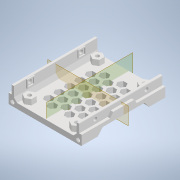
# Autodesk Inventor part: A-01
Saved by Autodesk Inventor 2022.2 (Build 262287000, 287)
## iProperties
Created: 2021-12-01
Part Number: A-01
Material: Generic
Document SubType Name: Modeling
Designer: kfcs7
Density: 1 g/cm^3
Appearance: Default
Author: kfcs7
Autodesk Inventor part; units mm, degrees
ref_plane "YZ Plane" through (0, 0, 0) normal (1, 0, 0) x (0, 1, 0)
ref_plane "XZ Plane" through (0, 0, 0) normal (0, 1, 0) x (-1, 0, 0)
ref_plane "XY Plane" through (0, 0, 0) normal (0, 0, 1) x (1, 0, 0)
sketch "Sketch1" plane through (0, 0, 0) normal (0, 1, 0) x (-1, 0, 0)
  line L0 (35, 40) -> (-35, 40)
  line L1 (-35, 40) -> (-35, -40)
  line L2 (-35, -40) -> (35, -40)
  line L3 (35, -40) -> (35, 40)
  line L4 (35, 40) -> (-35, -40) construction
  line L5 (-35, 40) -> (35, -40) construction
  point P0 (0, 0)
  dimension "d0" = 70
  dimension "d1" = 80
  constraints: 12 end point, 2 midpoint, 2 parallel, 1 horizontal, 1 perpendicular
  measures "d0" distance of L2.end L1.end
  measures "d1" distance of L1.end L0.end
extrude "Extrusion1" add sketch "Sketch1" along normal blind 17.5
chamfer "Chamfer1" distance 6 angle 45 2 edges at (35, 0, 0) (-35, 0, 0)
shell "Shell1" thickness 5 removed faces 3 at (9.6667, 11.6667, 40) at (-9.6667, 11.6667, -40) at (11.6667, 17.5, 13.3333)
ref_plane "Work Plane1" through (0, 17.5, -40) normal (-1, 0, 0) x (0, 0, 1)
ref_plane "Work Plane2" through (-29, 0, 0) normal (0, 0, 1) x (1, 0, 0)
sketch "Sketch2" plane through (-26.9289, 5, 40) normal (0, 1, 0) x (1, 0, 0)
  circle A0 centre (4.4289, 72.5) radius 1 construction
  circle A1 centre (49.4289, 72.5) radius 1 construction
  circle A2 centre (49.4289, 7.5) radius 1 construction
  circle A3 centre (4.4289, 7.5) radius 1 construction
  line L0 (1.9289, 75) -> (1.9289, 5) construction
  line L1 (1.9289, 5) -> (51.9289, 5) construction
  line L2 (51.9289, 5) -> (51.9289, 75) construction
  line L3 (51.9289, 75) -> (1.9289, 75) construction
  line L4 (4.4289, 67.3038) -> (-0.0711, 69.9019)
  line L5 (-0.0711, 69.9019) -> (-0.0711, 75.0981)
  line L6 (-0.0711, 75.0981) -> (4.4289, 77.6962)
  line L7 (4.4289, 77.6962) -> (8.9289, 75.0981)
  line L8 (8.9289, 75.0981) -> (8.9289, 69.9019)
  line L9 (8.9289, 69.9019) -> (4.4289, 67.3038)
  line L10 (44.9289, 69.9019) -> (44.9289, 75.0981)
  line L11 (44.9289, 75.0981) -> (49.4289, 77.6962)
  line L12 (49.4289, 77.6962) -> (53.9289, 75.0981)
  line L13 (53.9289, 75.0981) -> (53.9289, 69.9019)
  line L14 (53.9289, 69.9019) -> (49.4289, 67.3038)
  line L15 (49.4289, 67.3038) -> (44.9289, 69.9019)
  line L16 (4.4289, 12.6962) -> (8.9289, 10.0981)
  line L17 (8.9289, 10.0981) -> (8.9289, 4.9019)
  line L18 (8.9289, 4.9019) -> (4.4289, 2.3038)
  line L19 (4.4289, 2.3038) -> (-0.0711, 4.9019)
  line L20 (-0.0711, 4.9019) -> (-0.0711, 10.0981)
  line L21 (-0.0711, 10.0981) -> (4.4289, 12.6962)
  line L22 (44.9289, 10.0981) -> (49.4289, 12.6962)
  line L23 (49.4289, 12.6962) -> (53.9289, 10.0981)
  line L24 (53.9289, 10.0981) -> (53.9289, 4.9019)
  line L25 (53.9289, 4.9019) -> (49.4289, 2.3038)
  line L26 (49.4289, 2.3038) -> (44.9289, 4.9019)
  line L27 (44.9289, 4.9019) -> (44.9289, 10.0981)
  circle A4 centre (4.4289, 72.5) radius 1.25
  circle A5 centre (4.4289, 7.5) radius 1.25
  circle A6 centre (49.4289, 7.5) radius 1.25
  circle A7 centre (49.4289, 72.5) radius 1.25
  point P0 (26.9289, 40)
  dimension "d8" = 2.5
  dimension "d9" = 9
  dimension "d10" = 9
  dimension "d11" = 9
  dimension "d12" = 9
  dimension "d13" = 2.5
  dimension "d14" = 2.5
  dimension "d15" = 2.5
  constraints: 48 end point, 8 coincident, 4 centre point, 4 parallel, 52 other
  measures "d8" diameter of A4
  measures "d9" distance between parallel lines of L8 L5
  measures "d10" distance between parallel lines of L13 L10
  measures "d11" distance between parallel lines of L24 L27
  measures "d12" distance between parallel lines of L17 L20
  measures "d13" diameter of A5
  measures "d14" diameter of A6
  measures "d15" diameter of A7
extrude "Extrusion2" add sketch "Sketch2" along normal blind 5 draft -2.5 contours L4 L5 L6 L7 L8 L9 | L10 L11 L12 L13 L14 L15 | L16 L17 L18 L19 L20 L21 | L22 L23 L24 L25 L26 L27 | A4 | A5 | A6 | A7
sketch "Sketch3" plane through (-26.9289, 10, 40) normal (0, 1, 0) x (1, 0, 0)
  circle A0 centre (4.4289, 72.5) radius 1 construction
  circle A1 centre (49.4289, 72.5) radius 1 construction
  circle A2 centre (49.4289, 7.5) radius 1 construction
  circle A3 centre (4.4289, 7.5) radius 1 construction
  line L0 (1.9289, 75) -> (1.9289, 5) construction
  line L1 (1.9289, 5) -> (51.9289, 5) construction
  line L2 (51.9289, 5) -> (51.9289, 75) construction
  line L3 (51.9289, 75) -> (1.9289, 75) construction
  circle A4 centre (4.4289, 72.5) radius 1.5
  circle A5 centre (49.4289, 72.5) radius 1.5
  circle A6 centre (4.4289, 7.5) radius 1.5
  circle A7 centre (49.4289, 7.5) radius 1.5
  point P0 (26.9289, 40)
  dimension "d18" = 3
  constraints: 4 centre point, 4 coincident, 3 equal radius
  measures "d18" diameter of A4
extrude "Extrusion3" cut sketch "Sketch3" against normal blind 5 draft 2.5
fillet "Fillet1" radius 0.5 4 edges at (-24, 10, 32.5) (-24, 10, -32.5) (21, 10, -32.5) (21, 10, 32.5)
sketch "Sketch4" plane through (-26.9289, 5, 40) normal (0, 1, 0) x (1, 0, 0)
  line L0 (29.527, 35.5) -> (24.3309, 35.5)
  line L1 (24.3309, 35.5) -> (21.7328, 40)
  line L2 (21.7328, 40) -> (24.3309, 44.5)
  line L3 (24.3309, 44.5) -> (29.527, 44.5)
  line L4 (29.527, 44.5) -> (32.1251, 40)
  line L5 (32.1251, 40) -> (29.527, 35.5)
  line L6 (0, 80) -> (53.8579, 80) projected
  line L7 (28.9497, 43.5) -> (24.9082, 43.5)
  line L8 (24.9082, 43.5) -> (22.8875, 40)
  line L9 (22.8875, 40) -> (24.9082, 36.5)
  line L10 (24.9082, 36.5) -> (28.9497, 36.5)
  line L11 (28.9497, 36.5) -> (30.9704, 40)
  line L12 (30.9704, 40) -> (28.9497, 43.5)
  line L13 (13.9386, 44.5) -> (16.5366, 40)
  line L14 (16.5366, 40) -> (21.7328, 40)
  line L15 (24.3309, 44.5) -> (21.7328, 49)
  line L16 (21.7328, 49) -> (16.5366, 49)
  line L17 (16.5366, 49) -> (13.9386, 44.5)
  line L18 (21.1554, 48) -> (23.1762, 44.5)
  line L19 (23.1762, 44.5) -> (21.1554, 41)
  line L20 (21.1554, 41) -> (17.114, 41)
  line L21 (17.114, 41) -> (15.0933, 44.5)
  line L22 (15.0933, 44.5) -> (17.114, 48)
  line L23 (17.114, 48) -> (21.1554, 48)
  line L24 (29.527, 35.5) -> (32.1251, 31)
  line L25 (32.1251, 31) -> (37.3212, 31)
  line L26 (37.3212, 31) -> (39.9193, 35.5)
  line L27 (39.9193, 35.5) -> (37.3212, 40)
  line L28 (37.3212, 40) -> (32.1251, 40)
  line L29 (36.7439, 39) -> (38.7646, 35.5)
  line L30 (38.7646, 35.5) -> (36.7439, 32)
  line L31 (36.7439, 32) -> (32.7024, 32)
  line L32 (32.7024, 32) -> (30.6817, 35.5)
  line L33 (30.6817, 35.5) -> (32.7024, 39)
  line L34 (32.7024, 39) -> (36.7439, 39)
  line L35 (47.7135, 31) -> (45.1155, 26.5)
  line L36 (45.1155, 35.5) -> (47.7135, 31)
  line L37 (39.9193, 35.5) -> (45.1155, 35.5)
  line L38 (45.1155, 26.5) -> (39.9193, 26.5)
  line L39 (39.9193, 26.5) -> (37.3212, 31)
  line L40 (40.4967, 34.5) -> (38.4759, 31)
  line L41 (44.5381, 34.5) -> (40.4967, 34.5)
  line L42 (46.5588, 31) -> (44.5381, 34.5)
  line L43 (40.4967, 27.5) -> (44.5381, 27.5)
  line L44 (44.5381, 27.5) -> (46.5588, 31)
  line L45 (38.4759, 31) -> (40.4967, 27.5)
  line L46 (6.1443, 49) -> (8.7424, 53.5)
  line L47 (13.9386, 44.5) -> (8.7424, 44.5)
  line L48 (8.7424, 44.5) -> (6.1443, 49)
  line L49 (8.7424, 53.5) -> (13.9386, 53.5)
  line L50 (13.9386, 53.5) -> (16.5366, 49)
  line L51 (13.3612, 52.5) -> (9.3197, 52.5)
  line L52 (9.3197, 52.5) -> (7.299, 49)
  line L53 (7.299, 49) -> (9.3197, 45.5)
  line L54 (9.3197, 45.5) -> (13.3612, 45.5)
  line L55 (13.3612, 45.5) -> (15.3819, 49)
  line L56 (15.3819, 49) -> (13.3612, 52.5)
  point P0 (26.9289, 40)
  point P1 (26.9289, 40)
  point P2 (19.1347, 44.5)
  point P3 (19.1347, 44.5)
  point P4 (34.7232, 35.5)
  point P5 (34.7232, 35.5)
  point P6 (48.2909, 30)
  point P7 (42.5174, 31)
  point P8 (42.5174, 31)
  point P9 (5.567, 50)
  point P10 (11.3405, 49)
  point P11 (11.3405, 49)
  dimension "d22" = 9
  dimension "d23" = 1
  constraints: 112 end point, 52 symmetric about line, 5 coincident, 1 parallel, 18 other
  measures "d22" distance between parallel lines of L3 L0
  measures "d23" distance between parallel lines of L3 L7
extrude "Extrusion4" cut sketch "Sketch4" against normal through all contours L12 L11 L10 L9 L8 L7 | L18 L19 L20 L21 L22 L23 | L29 L30 L31 L32 L33 L34 | L41 L42 L44 L43 L45 L40 | L56 L55 L54 L53 L52 L51
pattern_linear "Rectangular Pattern1" count 7 spacing 10 along (0, 0, -1) of "Extrusion4" first direction both ways yes
sketch "Sketch7" plane through (0, 0, 0) normal (0, -1, 0) x (1, 0, 0)
  line L0 (-11.547, -39) -> (-12.1244, -40) projected
  line L1 (29, -40) -> (-12.1244, -40) projected
  line L2 (29, 40) -> (29, -40) projected
  line L3 (19.0526, 40) -> (29, 40) projected
  line L4 (19.0526, 40) -> (19.6299, 39) projected
  line L5 (19.6299, 39) -> (17.6092, 35.5) projected
  line L6 (17.6092, 35.5) -> (13.5677, 35.5) projected
  line L7 (13.5677, 35.5) -> (11.547, 39) projected
  line L8 (11.547, 39) -> (12.1244, 40) projected
  line L9 (-29, 40) -> (12.1244, 40) projected
  line L10 (-29, -40) -> (-29, 40) projected
  line L11 (-19.0526, -40) -> (-29, -40) projected
  line L12 (-19.0526, -40) -> (-19.6299, -39) projected
  line L13 (-19.6299, -39) -> (-17.6092, -35.5) projected
  line L14 (-17.6092, -35.5) -> (-13.5677, -35.5) projected
  line L15 (-13.5677, -35.5) -> (-11.547, -39) projected
  line L16 (9.815, -22) -> (11.8357, -25.5) projected
  line L17 (11.8357, -25.5) -> (9.815, -29) projected
  line L18 (9.815, -29) -> (5.7735, -29) projected
  line L19 (5.7735, -29) -> (3.7528, -25.5) projected
  line L20 (3.7528, -25.5) -> (5.7735, -22) projected
  line L21 (5.7735, -22) -> (9.815, -22) projected
  line L22 (-5.7735, -31) -> (-3.7528, -34.5) projected
  line L23 (-3.7528, -34.5) -> (-5.7735, -38) projected
  line L24 (-5.7735, -38) -> (-9.815, -38) projected
  line L25 (-9.815, -38) -> (-11.8357, -34.5) projected
  line L26 (-11.8357, -34.5) -> (-9.815, -31) projected
  line L27 (-9.815, -31) -> (-5.7735, -31) projected
  line L28 (13.5677, -17.5) -> (17.6092, -17.5) projected
  line L29 (17.6092, -17.5) -> (19.6299, -21) projected
  line L30 (19.6299, -21) -> (17.6092, -24.5) projected
  line L31 (17.6092, -24.5) -> (13.5677, -24.5) projected
  line L32 (13.5677, -24.5) -> (11.547, -21) projected
  line L33 (11.547, -21) -> (13.5677, -17.5) projected
  line L34 (2.0207, -26.5) -> (4.0415, -30) projected
  line L35 (4.0415, -30) -> (2.0207, -33.5) projected
  line L36 (2.0207, -33.5) -> (-2.0207, -33.5) projected
  line L37 (-2.0207, -33.5) -> (-4.0415, -30) projected
  line L38 (-4.0415, -30) -> (-2.0207, -26.5) projected
  line L39 (-2.0207, -26.5) -> (2.0207, -26.5) projected
  line L40 (9.815, -12) -> (11.8357, -15.5) projected
  line L41 (11.8357, -15.5) -> (9.815, -19) projected
  line L42 (9.815, -19) -> (5.7735, -19) projected
  line L43 (5.7735, -19) -> (3.7528, -15.5) projected
  line L44 (3.7528, -15.5) -> (5.7735, -12) projected
  line L45 (5.7735, -12) -> (9.815, -12) projected
  line L46 (-19.6299, -29) -> (-17.6092, -25.5) projected
  line L47 (-17.6092, -25.5) -> (-13.5677, -25.5) projected
  line L48 (-13.5677, -25.5) -> (-11.547, -29) projected
  line L49 (-11.547, -29) -> (-13.5677, -32.5) projected
  line L50 (-13.5677, -32.5) -> (-17.6092, -32.5) projected
  line L51 (-17.6092, -32.5) -> (-19.6299, -29) projected
  line L52 (-5.7735, -21) -> (-3.7528, -24.5) projected
  line L53 (-3.7528, -24.5) -> (-5.7735, -28) projected
  line L54 (-5.7735, -28) -> (-9.815, -28) projected
  line L55 (-9.815, -28) -> (-11.8357, -24.5) projected
  line L56 (-11.8357, -24.5) -> (-9.815, -21) projected
  line L57 (-9.815, -21) -> (-5.7735, -21) projected
  line L58 (13.5677, -7.5) -> (17.6092, -7.5) projected
  line L59 (17.6092, -7.5) -> (19.6299, -11) projected
  line L60 (19.6299, -11) -> (17.6092, -14.5) projected
  line L61 (17.6092, -14.5) -> (13.5677, -14.5) projected
  line L62 (13.5677, -14.5) -> (11.547, -11) projected
  line L63 (11.547, -11) -> (13.5677, -7.5) projected
  line L64 (2.0207, -16.5) -> (4.0415, -20) projected
  line L65 (4.0415, -20) -> (2.0207, -23.5) projected
  line L66 (2.0207, -23.5) -> (-2.0207, -23.5) projected
  line L67 (-2.0207, -23.5) -> (-4.0415, -20) projected
  line L68 (-4.0415, -20) -> (-2.0207, -16.5) projected
  line L69 (-2.0207, -16.5) -> (2.0207, -16.5) projected
  line L70 (9.815, -2) -> (11.8357, -5.5) projected
  line L71 (11.8357, -5.5) -> (9.815, -9) projected
  line L72 (9.815, -9) -> (5.7735, -9) projected
  line L73 (5.7735, -9) -> (3.7528, -5.5) projected
  line L74 (3.7528, -5.5) -> (5.7735, -2) projected
  line L75 (5.7735, -2) -> (9.815, -2) projected
  line L76 (-19.6299, -19) -> (-17.6092, -15.5) projected
  line L77 (-17.6092, -15.5) -> (-13.5677, -15.5) projected
  line L78 (-13.5677, -15.5) -> (-11.547, -19) projected
  line L79 (-11.547, -19) -> (-13.5677, -22.5) projected
  line L80 (-13.5677, -22.5) -> (-17.6092, -22.5) projected
  line L81 (-17.6092, -22.5) -> (-19.6299, -19) projected
  line L82 (-5.7735, -11) -> (-3.7528, -14.5) projected
  line L83 (-3.7528, -14.5) -> (-5.7735, -18) projected
  line L84 (-5.7735, -18) -> (-9.815, -18) projected
  line L85 (-9.815, -18) -> (-11.8357, -14.5) projected
  line L86 (-11.8357, -14.5) -> (-9.815, -11) projected
  line L87 (-9.815, -11) -> (-5.7735, -11) projected
  line L88 (13.5677, 2.5) -> (17.6092, 2.5) projected
  line L89 (17.6092, 2.5) -> (19.6299, -1) projected
  line L90 (19.6299, -1) -> (17.6092, -4.5) projected
  line L91 (17.6092, -4.5) -> (13.5677, -4.5) projected
  line L92 (13.5677, -4.5) -> (11.547, -1) projected
  line L93 (11.547, -1) -> (13.5677, 2.5) projected
  line L94 (2.0207, -6.5) -> (4.0415, -10) projected
  line L95 (4.0415, -10) -> (2.0207, -13.5) projected
  line L96 (2.0207, -13.5) -> (-2.0207, -13.5) projected
  line L97 (-2.0207, -13.5) -> (-4.0415, -10) projected
  line L98 (-4.0415, -10) -> (-2.0207, -6.5) projected
  line L99 (-2.0207, -6.5) -> (2.0207, -6.5) projected
  line L100 (9.815, 18) -> (11.8357, 14.5) projected
  line L101 (11.8357, 14.5) -> (9.815, 11) projected
  line L102 (9.815, 11) -> (5.7735, 11) projected
  line L103 (5.7735, 11) -> (3.7528, 14.5) projected
  line L104 (3.7528, 14.5) -> (5.7735, 18) projected
  line L105 (5.7735, 18) -> (9.815, 18) projected
  line L106 (-19.6299, 1) -> (-17.6092, 4.5) projected
  line L107 (-17.6092, 4.5) -> (-13.5677, 4.5) projected
  line L108 (-13.5677, 4.5) -> (-11.547, 1) projected
  line L109 (-11.547, 1) -> (-13.5677, -2.5) projected
  line L110 (-13.5677, -2.5) -> (-17.6092, -2.5) projected
  line L111 (-17.6092, -2.5) -> (-19.6299, 1) projected
  line L112 (-5.7735, 9) -> (-3.7528, 5.5) projected
  line L113 (-3.7528, 5.5) -> (-5.7735, 2) projected
  line L114 (-5.7735, 2) -> (-9.815, 2) projected
  line L115 (-9.815, 2) -> (-11.8357, 5.5) projected
  line L116 (-11.8357, 5.5) -> (-9.815, 9) projected
  line L117 (-9.815, 9) -> (-5.7735, 9) projected
  line L118 (13.5677, 22.5) -> (17.6092, 22.5) projected
  line L119 (17.6092, 22.5) -> (19.6299, 19) projected
  line L120 (19.6299, 19) -> (17.6092, 15.5) projected
  line L121 (17.6092, 15.5) -> (13.5677, 15.5) projected
  line L122 (13.5677, 15.5) -> (11.547, 19) projected
  line L123 (11.547, 19) -> (13.5677, 22.5) projected
  line L124 (2.0207, 13.5) -> (4.0415, 10) projected
  line L125 (4.0415, 10) -> (2.0207, 6.5) projected
  line L126 (2.0207, 6.5) -> (-2.0207, 6.5) projected
  line L127 (-2.0207, 6.5) -> (-4.0415, 10) projected
  line L128 (-4.0415, 10) -> (-2.0207, 13.5) projected
  line L129 (-2.0207, 13.5) -> (2.0207, 13.5) projected
  line L130 (9.815, 28) -> (11.8357, 24.5) projected
  line L131 (11.8357, 24.5) -> (9.815, 21) projected
  line L132 (9.815, 21) -> (5.7735, 21) projected
  line L133 (5.7735, 21) -> (3.7528, 24.5) projected
  line L134 (3.7528, 24.5) -> (5.7735, 28) projected
  line L135 (5.7735, 28) -> (9.815, 28) projected
  line L136 (-19.6299, 11) -> (-17.6092, 14.5) projected
  line L137 (-17.6092, 14.5) -> (-13.5677, 14.5) projected
  line L138 (-13.5677, 14.5) -> (-11.547, 11) projected
  line L139 (-11.547, 11) -> (-13.5677, 7.5) projected
  line L140 (-13.5677, 7.5) -> (-17.6092, 7.5) projected
  line L141 (-17.6092, 7.5) -> (-19.6299, 11) projected
  line L142 (-5.7735, 19) -> (-3.7528, 15.5) projected
  line L143 (-3.7528, 15.5) -> (-5.7735, 12) projected
  line L144 (-5.7735, 12) -> (-9.815, 12) projected
  line L145 (-9.815, 12) -> (-11.8357, 15.5) projected
  line L146 (-11.8357, 15.5) -> (-9.815, 19) projected
  line L147 (-9.815, 19) -> (-5.7735, 19) projected
  line L148 (13.5677, 32.5) -> (17.6092, 32.5) projected
  line L149 (17.6092, 32.5) -> (19.6299, 29) projected
  line L150 (19.6299, 29) -> (17.6092, 25.5) projected
  line L151 (17.6092, 25.5) -> (13.5677, 25.5) projected
  line L152 (13.5677, 25.5) -> (11.547, 29) projected
  line L153 (11.547, 29) -> (13.5677, 32.5) projected
  line L154 (2.0207, 23.5) -> (4.0415, 20) projected
  line L155 (4.0415, 20) -> (2.0207, 16.5) projected
  line L156 (2.0207, 16.5) -> (-2.0207, 16.5) projected
  line L157 (-2.0207, 16.5) -> (-4.0415, 20) projected
  line L158 (-4.0415, 20) -> (-2.0207, 23.5) projected
  line L159 (-2.0207, 23.5) -> (2.0207, 23.5) projected
  line L160 (9.815, 38) -> (11.8357, 34.5) projected
  line L161 (11.8357, 34.5) -> (9.815, 31) projected
  line L162 (9.815, 31) -> (5.7735, 31) projected
  line L163 (5.7735, 31) -> (3.7528, 34.5) projected
  line L164 (3.7528, 34.5) -> (5.7735, 38) projected
  line L165 (5.7735, 38) -> (9.815, 38) projected
  line L166 (-19.6299, 21) -> (-17.6092, 24.5) projected
  line L167 (-17.6092, 24.5) -> (-13.5677, 24.5) projected
  line L168 (-13.5677, 24.5) -> (-11.547, 21) projected
  line L169 (-11.547, 21) -> (-13.5677, 17.5) projected
  line L170 (-13.5677, 17.5) -> (-17.6092, 17.5) projected
  line L171 (-17.6092, 17.5) -> (-19.6299, 21) projected
  line L172 (-5.7735, 29) -> (-3.7528, 25.5) projected
  line L173 (-3.7528, 25.5) -> (-5.7735, 22) projected
  line L174 (-5.7735, 22) -> (-9.815, 22) projected
  line L175 (-9.815, 22) -> (-11.8357, 25.5) projected
  line L176 (-11.8357, 25.5) -> (-9.815, 29) projected
  line L177 (-9.815, 29) -> (-5.7735, 29) projected
  line L178 (2.0207, 33.5) -> (4.0415, 30) projected
  line L179 (4.0415, 30) -> (2.0207, 26.5) projected
  line L180 (2.0207, 26.5) -> (-2.0207, 26.5) projected
  line L181 (-2.0207, 26.5) -> (-4.0415, 30) projected
  line L182 (-4.0415, 30) -> (-2.0207, 33.5) projected
  line L183 (-2.0207, 33.5) -> (2.0207, 33.5) projected
  line L184 (5.7735, 1) -> (3.7528, 4.5) projected
  line L185 (3.7528, 4.5) -> (5.7735, 8) projected
  line L186 (5.7735, 8) -> (9.815, 8) projected
  line L187 (9.815, 8) -> (11.8357, 4.5) projected
  line L188 (11.8357, 4.5) -> (9.815, 1) projected
  line L189 (9.815, 1) -> (5.7735, 1) projected
  line L190 (-4.0415, 0) -> (-2.0207, 3.5) projected
  line L191 (-2.0207, 3.5) -> (2.0207, 3.5) projected
  line L192 (2.0207, 3.5) -> (4.0415, 0) projected
  line L193 (4.0415, 0) -> (2.0207, -3.5) projected
  line L194 (2.0207, -3.5) -> (-2.0207, -3.5) projected
  line L195 (-2.0207, -3.5) -> (-4.0415, 0) projected
  line L196 (17.6092, 5.5) -> (13.5677, 5.5) projected
  line L197 (13.5677, 5.5) -> (11.547, 9) projected
  line L198 (11.547, 9) -> (13.5677, 12.5) projected
  line L199 (13.5677, 12.5) -> (17.6092, 12.5) projected
  line L200 (17.6092, 12.5) -> (19.6299, 9) projected
  line L201 (19.6299, 9) -> (17.6092, 5.5) projected
  line L202 (-11.8357, -4.5) -> (-9.815, -1) projected
  line L203 (-9.815, -1) -> (-5.7735, -1) projected
  line L204 (-5.7735, -1) -> (-3.7528, -4.5) projected
  line L205 (-3.7528, -4.5) -> (-5.7735, -8) projected
  line L206 (-5.7735, -8) -> (-9.815, -8) projected
  line L207 (-9.815, -8) -> (-11.8357, -4.5) projected
  line L208 (-11.547, -9) -> (-13.5677, -12.5) projected
  line L209 (-13.5677, -12.5) -> (-17.6092, -12.5) projected
  line L210 (-17.6092, -12.5) -> (-19.6299, -9) projected
  line L211 (-19.6299, -9) -> (-17.6092, -5.5) projected
  line L212 (-17.6092, -5.5) -> (-13.5677, -5.5) projected
  line L213 (-13.5677, -5.5) -> (-11.547, -9) projected
  line L214 (29, -40) -> (-12.1244, -40) projected
  line L215 (-12.1244, -40) -> (-19.0526, -40)
  line L216 (19.0526, 40) -> (19.6299, 39) projected
  line L217 (11.547, 39) -> (12.1244, 40) projected
  line L218 (19.0526, 40) -> (12.1244, 40)
  point P0 (0, 0)
  constraints: 4 end point, 1 horizontal
extrude "Extrusion7" add sketch "Sketch7" against normal up to surface (5 mm away) contours L0 L215 L12 L13 L14 L15 | L4 L5 L6 L7 L8 L218 | L22 L23 L24 L25 L26 L27 | L34 L35 L36 L37 L38 L39 | L46 L47 L48 L49 L50 L51 | L148 L149 L150 L151 L152 L153 | L160 L161 L162 L163 L164 L165 | L178 L179 L180 L181 L182 L183
sketch "Sketch6" plane through (35, 17.5, 40) normal (1, 0, 0) x (0, 0, -1)
  line L0 (80, -11.5) -> (0, -11.5) projected
  line L1 (80, -11.5) -> (80, 0) projected
  line L2 (0, 0) -> (80, 0) projected
  line L3 (0, -11.5) -> (0, 0) projected
  line L4 (0, 0) -> (0, -9.4289) projected
  line L5 (0, -8) -> (80, -8)
  point P0 (40, -17.5)
  dimension "d31" = 8
  constraints: 2 end point, 2 point on line, 1 perpendicular
  measures "d31" distance between parallel lines of L2 L5
extrude "Extrusion6" cut sketch "Sketch6" against normal blind 2.5 contours L5 L3 L2 L1
fillet "Fillet2" radius 0.5 3 edges at (32.5, 13.5, -40) (32.5, 13.5, 40) (32.5, 17.5, 0)
sketch "Sketch8" plane through (32.5, 17.5, 40) normal (1, 0, 0) x (0, 0, -1)
  line L0 (79.5, -0.5) -> (79.5, -8) projected
  line L1 (0.5, -0.5) -> (79.5, -0.5) projected
  line L2 (0.5, -8) -> (0.5, -0.5) projected
  line L3 (79.5, -8) -> (0.5, -8) projected
  circle A0 centre (15.4979, -4) radius 1.75
  line L4 (80, 0) -> (0, 0) projected
  line L5 (0, 0) -> (0, -8) projected
  point P0 (40, -17.5)
  point P1 (0.5, -4.25)
  dimension "d37" = 15
  dimension "d38" = 3.5
  dimension "d40" = 4
  dimension "d41" = 8
  constraints: 1 centre point, 1 midpoint
  measures "d37" distance of point (0.5, -4.25) A0.centre
  measures "d38" diameter of A0
  measures "d40" distance from line of L4 A0.centre
  measures "d41" distance of L4.end L5.end
extrude "Extrusion8" cut sketch "Sketch8" against normal up to surface (2.5 mm away) contours A0
sketch "Sketch9" plane through (30, 8.0711, 40) normal (-1, 0, 0) x (0, 0, 1)
  circle A0 centre (-15.4979, 5.4289) radius 1.75 construction
  line L0 (-18.2479, 8.1789) -> (-12.7479, 8.1789)
  line L1 (-12.7479, 8.1789) -> (-12.7479, 2.6789)
  line L2 (-12.7479, 2.6789) -> (-18.2479, 2.6789)
  line L3 (-18.2479, 2.6789) -> (-18.2479, 8.1789)
  line L4 (-18.2479, 8.1789) -> (-12.7479, 2.6789) construction
  line L5 (-12.7479, 8.1789) -> (-18.2479, 2.6789) construction
  line L6 (-11.7479, 9.1789) -> (-19.2479, 9.1789)
  line L7 (-19.2479, 9.1789) -> (-19.2479, 1.6789)
  line L8 (-19.2479, 1.6789) -> (-11.7479, 1.6789)
  line L9 (-11.7479, 1.6789) -> (-11.7479, 9.1789)
  point P0 (-40, -8.0711)
  dimension "d44" = 5.5
  dimension "d45" = 5.5
  dimension "d46" = 1
  constraints: 20 end point, 4 parallel, 2 midpoint, 2 perpendicular, 1 horizontal, 3 other
  measures "d44" distance of L1.end L2.end
  measures "d45" distance of L0.end L1.end
  measures "d46" distance between parallel lines of L0 L6
extrude "Extrusion9" add sketch "Sketch9" along normal blind 1
chamfer "Chamfer2" distance 0.5 angle 45 4 edges at (29.5, 9.75, 28.2521) (29.5, 17.25, 28.2521) (29.5, 17.25, 20.7521) (29.5, 9.75, 20.7521)
mirror "Mirror1" about plane through (-29, 0, 0) normal (0, 0, 1) of "Extrusion8", "Extrusion9", "Chamfer2"
sketch "Sketch13" plane through (35, 6, 40) normal (1, 0, 0) x (0, 0, -1)
  circle A0 centre (15.4979, 7.5) radius 1.75 construction
  circle A1 centre (64.5021, 7.5) radius 1.75 construction
  line L0 (15.4979, 7.5) -> (64.5021, 7.5) construction
  line L1 (79.5, 3.5) -> (0.5, 3.5) projected
  line L2 (27.1992, 3.5) -> (30, 7.5)
  line L3 (50, 7.5) -> (52.8008, 3.5)
  line L4 (50, 7.5) -> (30, 7.5)
  point P0 (40, -6)
  point P1 (40, 7.5)
  dimension "d65" = 10
  dimension "d66" = 20
  dimension "d67" = 125
  dimension "d68" = 125
  constraints: 8 end point, 4 point on line, 1 collinear, 1 horizontal, 1 midpoint
  measures "d65" distance of L3.start point (40, 7.5)
  measures "d66" distance of L3.start L2.end
  measures "d67" angle of L0 L3
  measures "d68" angle of L0 L2
extrude "Extrusion13" add sketch "Sketch13" against normal up to surface (2.5 mm away)
mirror "Mirror2" about plane through (0, 17.5, -40) normal (-1, 0, 0) of "Extrusion6", "Extrusion8", "Extrusion9", "Mirror1", "Fillet2", "Extrusion13"
sketch "Sketch10" plane through (-29, 0, 40) normal (0, 0, 1) x (1, 0, 0)
  line L0 (-3, 9.5) -> (-3, 17.5) projected
  line L1 (-3, 9.5) -> (-6, 9.5) projected
  line L2 (-6, 6) -> (-6, 9.5) projected
  line L3 (0, 0) -> (-6, 6) projected
  line L4 (0, 0) -> (58, 0) projected
  line L5 (64, 6) -> (58, 0) projected
  line L6 (64, 6) -> (64, 9.5) projected
  line L7 (64, 9.5) -> (61, 9.5) projected
  line L8 (61, 17.5) -> (61, 9.5) projected
  line L9 (59, 17.5) -> (61, 17.5) projected
  line L10 (59, 17.5) -> (59, 8.0711) projected
  line L11 (59, 8.0711) -> (55.9289, 5) projected
  line L12 (55.9289, 5) -> (2.0711, 5) projected
  line L13 (2.0711, 5) -> (-1, 8.0711) projected
  line L14 (-1, 8.0711) -> (-1, 17.5) projected
  line L15 (-3, 17.5) -> (-1, 17.5) projected
  line L16 (0, 0) -> (-6, 6) projected
  line L17 (-6, 6) -> (-6, 0)
  line L18 (-6, 0) -> (0, 0)
  point P0 (29, 0)
  constraints: 4 end point, 1 perpendicular, 1 point on line
extrude "Extrusion10" add sketch "Sketch10" against normal blind 20 contours L3 L18 L17
sketch "Sketch11" plane through (-35, 0, 40) normal (-1, 0, 0) x (0, 0, 1)
  line L0 (0, 9.5) -> (-27.1992, 9.5) projected
  line L1 (-80, 6) -> (-80, 9.5) projected
  line L2 (-20, 6) -> (-80, 6) projected
  line L3 (-20, 0) -> (-20, 6) projected
  line L4 (0, 0) -> (-20, 0) projected
  line L5 (0, 0) -> (0, 9.5) projected
  line L6 (-20, 0) -> (-20, 6) projected
  line L7 (-20, 6) -> (-14.9654, 0)
  line L8 (-15.5, 0) -> (-19, 0) projected
  line L9 (-20, 6) -> (-12.1676, 6) construction
  line L10 (-30, 13.5) -> (-27.1992, 9.5) projected
  line L11 (-50, 13.5) -> (-30, 13.5) projected
  line L12 (-52.8008, 9.5) -> (-50, 13.5) projected
  line L13 (-52.8008, 9.5) -> (-80, 9.5) projected
  point P0 (-40, 0)
  point P1 (-14.9654, 0)
  dimension "d54" = 50
  constraints: 4 end point, 1 equal length, 1 horizontal, 1 point on line
  measures "d54" angle of L7 L9
extrude "Extrusion11" cut sketch "Sketch11" against normal up to surface contours L4 L3 L7 surface through (-32, 3, -20) normal (-0.7071068, -0.7071068, 0)
sketch "Sketch12" plane through (-35, 0, 40) normal (0, 0, 1) x (1, 0, 0)
  line L0 (3, 9.5) -> (3, 17.5) projected
  line L1 (3, 9.5) -> (0, 9.5) projected
  line L2 (0, 0) -> (0, 9.5) projected
  line L3 (0, 0) -> (64, 0) projected
  line L4 (70, 6) -> (64, 0) projected
  line L5 (70, 6) -> (70, 9.5) projected
  line L6 (70, 9.5) -> (67, 9.5) projected
  line L7 (67, 17.5) -> (67, 9.5) projected
  line L8 (65, 17.5) -> (67, 17.5) projected
  line L9 (65, 17.5) -> (65, 8.0711) projected
  line L10 (65, 8.0711) -> (61.9289, 5) projected
  line L11 (61.9289, 5) -> (8.0711, 5) projected
  line L12 (8.0711, 5) -> (5, 8.0711) projected
  line L13 (5, 8.0711) -> (5, 17.5) projected
  line L14 (3, 17.5) -> (5, 17.5) projected
  line L15 (8.0711, 5) -> (5, 8.0711) projected
  line L16 (0, 0) -> (64, 0) projected
  line L17 (6.5355, 6.5355) -> (0, 0)
  circle A0 centre (3.5355, 3.5355) radius 1.5
  point P0 (35, 0)
  dimension "d57" = 5
  dimension "d58" = 3
  constraints: 2 end point, 1 centre point, 1 midpoint, 1 point on line
  measures "d57" distance of L2.start A0.centre
  measures "d58" diameter of A0
extrude "Extrusion12" cut sketch "Sketch12" against normal blind 5 draft 2.5 contours A0 L17 | L17 A0
mirror "Mirror3" about plane through (-29, 0, 0) normal (0, 0, 1) of "Extrusion12", "Extrusion11", "Extrusion10"
mirror "Mirror4" about plane through (0, 17.5, -40) normal (-1, 0, 0) of "Extrusion12", "Extrusion11", "Extrusion10", "Mirror3"
chamfer "Chamfer4" distance 0.5 angle 45 8 edges at (-32.9645, 3.5355, -40) (-35, 0, -32.5173) (-35, 0, 32.5173) (-32.9645, 3.5355, 40) (35, 0, 32.5173) (35, 0, -32.5173) (32.9645, 3.5355, -40) (32.9645, 3.5355, 40)
equation "\"d10\" = d9"
equation "\"d11\" = d9"
equation "\"d12\" = d9"
equation "\"d40\" = 0.5 * d41"
equation "\"d45\" = d44"
equation "\"d65\" = 0.5 * d66"
body "Solid1"
